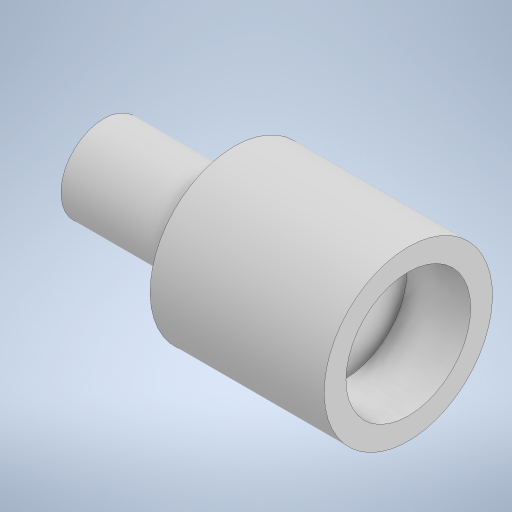
# Autodesk Inventor part: MagHolder
Saved by Autodesk Inventor 2024 (Build 280153000, 153)
## iProperties
Created: 2023-09-22
Part Number: MagHolder
Material: Generic
Document SubType Name: Modeling
Designer: RedStar
Density: 1 g/cm^3
Appearance: Default
Author: RedStar
Autodesk Inventor part; units mm, degrees
ref_plane "YZ Plane" through (0, 0, 0) normal (1, 0, 0) x (0, 1, 0)
ref_plane "XZ Plane" through (0, 0, 0) normal (0, 1, 0) x (-1, 0, 0)
ref_plane "XY Plane" through (0, 0, 0) normal (0, 0, 1) x (1, 0, 0)
sketch "Sketch1" plane through (0, 0, 0) normal (0, 0, 1) x (1, 0, 0)
  line L0 (-2.2, 0) -> (-2.2, 2.15)
  line L1 (-2.2, 2.15) -> (0, 2.15)
  line L2 (0, 2.15) -> (0, 2.9)
  line L3 (0, 2.9) -> (-6, 2.9)
  line L4 (-6, 2.9) -> (-6, 1.475)
  line L5 (-6, 1.475) -> (-10.5, 1.475)
  line L6 (-10.5, 1.475) -> (-10.5, 0)
  line L7 (-10.5, 0) -> (-2.2, 0)
  point P0 (0, 0)
  point P1 (-6.35, 0)
  point P2 (0, 2.525)
  dimension "d0" = 5.8
  dimension "d2" = 4.3
  dimension "d3" = 2.2
  dimension "d4" = 4.5
  dimension "d6" = 2.95
  dimension "d7" = 6
  constraints: 16 end point, 7 perpendicular, 2 midpoint, 1 horizontal alignment, 1 vertical, 1 vertical alignment
  measures "d0" diameter of L3 L7
  measures "d2" diameter of L1 L7
  measures "d3" distance from line of point (0, 0) L0
  measures "d4" distance between parallel lines of L4 L6
  measures "d6" diameter of L5 L7
  measures "d7" distance from line of point (0, 0) L4
revolve "Revolution1" add sketch "Sketch1" angle 360 about axis through (-10.5, 0, 0) along (1, 0, 0)
body "Solid1"
